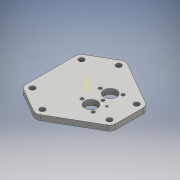
# Autodesk Inventor part: efector
Saved by Autodesk Inventor 2016 SP1 (Build 200210100, 210)
## iProperties
Created: 2016-03-06
Part Number: efector
Material: Generic
Document SubType Name: Modeling
Designer: roduino
Density: 1 g/cm^3
Appearance: Default
Author: roduino
Autodesk Inventor part; units mm, degrees
ref_plane "YZ Plane" through (0, 0, 0) normal (1, 0, 0) x (0, 1, 0)
ref_plane "XZ Plane" through (0, 0, 0) normal (0, 1, 0) x (-1, 0, 0)
ref_plane "XY Plane" through (0, 0, 0) normal (0, 0, 1) x (1, 0, 0)
sketch "Sketch1" plane through (0, 0, 0) normal (0, 0, 1) x (1, 0, 0)
  circle A0 centre (12.9186, 9) radius 6
  circle A1 centre (12.9186, -9) radius 6
  circle A2 centre (-28, 23) radius 2.5
  circle A3 centre (-28, -23) radius 2.5
  arc A4 (-31.4115, -18.0643) -> (-23.8208, -27.3051) centre (-28, -23) ccw
  arc A5 (-23.8208, 27.3051) -> (-31.4115, 18.0643) centre (-28, 23) ccw
  line L0 (-28, 23) -> (-28, -23) construction
  circle A6 centre (0, 0) radius 36.2353 construction
  arc A7 (-11.7365, -34.282) -> (0.0617, -36.2353) centre (-5.9186, -35.7487) ccw
  circle A8 centre (-5.9186, -35.7487) radius 2.5
  arc A9 (31.3499, -18.171) -> (35.5573, -6.9768) centre (33.9186, -12.7487) ccw
  circle A10 centre (33.9186, -12.7487) radius 2.5
  arc A11 (35.5573, 6.9768) -> (31.3499, 18.171) centre (33.9186, 12.7487) ccw
  circle A12 centre (33.9186, 12.7487) radius 2.5
  arc A13 (0.0617, 36.2353) -> (-11.7365, 34.282) centre (-5.9186, 35.7487) ccw
  circle A14 centre (-5.9186, 35.7487) radius 2.5
  line L1 (33.9186, 12.7487) -> (33.9186, -12.7487) construction
  line L2 (-34, 23) -> (-34, -23)
  line L3 (39.9186, 12.7487) -> (39.9186, -12.7487)
  line L4 (-31, 28.1962) -> (-8.9186, 40.9449)
  line L5 (-2.9186, 40.9449) -> (36.9186, 17.9449)
  line L6 (36.9186, -17.9449) -> (-2.9186, -40.9449)
  line L7 (-31, -28.1962) -> (-8.9186, -40.9449)
  dimension "d0" = 12
  dimension "d1" = 12
  dimension "d4" = 5
  dimension "d5" = 5
  dimension "d6" = 46
  dimension "d7" = 23
  dimension "d8" = 28
  dimension "d9" = 28
  dimension "d10" = 12
  dimension "d11" = 12
  dimension "d15" = 360
  dimension "d42" = 25.4974
  dimension "d43" = 27
  dimension "d44" = 27
  dimension "d45" = 9
  dimension "d46" = 9
  constraints: 29 point on circle, 16 end point, 15 centre point, 8 tangent, 7 coincident, 3 parallel, 1 vertical, 37 other
  measures "d0" diameter of A0
  measures "d1" diameter of A1
  measures "d4" diameter of A2
  measures "d5" diameter of A3
  measures "d6" distance of A3.centre A2.centre
  measures "d7" vertical distance of point (0, 0) A3.centre
  measures "d8" horizontal distance of point (0, 0) A2.centre
  measures "d9" horizontal distance of point (0, 0) A3.centre
  measures "d10" diameter of A4
  measures "d11" diameter of A5
  measures "d42" distance of A9.centre A11.centre
  measures "d43" distance from line of L3 A0.centre
  measures "d44" distance from line of L3 A1.centre
  measures "d45" vertical distance of point (0, 0) A0.centre
  measures "d46" vertical distance of point (0, 0) A1.centre
extrude "Extrusion1" add sketch "Sketch1" along normal blind 5
sketch "Sketch2" plane through (0, 0, 5) normal (0, 0, 1) x (1, 0, 0)
  circle A0 centre (12.9186, 9) radius 6 projected
  circle A1 centre (12.9186, -9) radius 6 projected
  circle A2 centre (15, 0) radius 1.5
  circle A3 centre (4, 8.5) radius 1.5
  circle A4 centre (4, -8.5) radius 1.5
  point P0 (0, 0)
  dimension "d19" = 3
  dimension "d20" = 3
  dimension "d21" = 3
  dimension "d22" = 15
  dimension "d25" = 17
  dimension "d26" = 8.5
  dimension "d47" = 4
  dimension "d48" = 4
  constraints: 3 centre point
  measures "d19" diameter of A2
  measures "d20" diameter of A3
  measures "d21" diameter of A4
  measures "d22" distance of point (0, 0) A2.centre
  measures "d25" distance of A4.centre A3.centre
  measures "d26" vertical distance of point (0, 0) A3.centre
  measures "d47" horizontal distance of point (0, 0) A3.centre
  measures "d48" horizontal distance of point (0, 0) A4.centre
extrude "Extrusion2" cut sketch "Sketch2" against normal through all contours A2 | A3 | A4
sketch "Sketch3" plane through (0, 0, 5) normal (0, 0, 1) x (1, 0, 0)
  circle A0 centre (20, 14) radius 1.5
  circle A1 centre (20, -14) radius 1.5
  point P0 (0, 0)
  dimension "d29" = 3
  dimension "d30" = 3
  dimension "d31" = 28
  dimension "d32" = 20
  dimension "d33" = 14
  dimension "d34" = 20
  constraints: 2 centre point
  measures "d29" diameter of A0
  measures "d30" diameter of A1
  measures "d31" distance of A1.centre A0.centre
  measures "d32" horizontal distance of point (0, 0) A1.centre
  measures "d33" vertical distance of point (0, 0) A1.centre
  measures "d34" horizontal distance of point (0, 0) A0.centre
extrude "Extrusion3" cut sketch "Sketch3" against normal through all
sketch "Sketch6" plane through (0, 0, 5) normal (0, 0, 1) x (1, 0, 0)
  arc A0 (22.75, -18) -> (24.75, -16) centre (22.75, -16) ccw projected
  line L0 (22.75, -18) -> (17.25, -18) projected
  arc A1 (15.25, -16) -> (17.25, -18) centre (17.25, -16) ccw projected
  line L1 (15.25, -16) -> (15.25, 16) projected
  arc A2 (17.25, 18) -> (15.25, 16) centre (17.25, 16) ccw projected
  line L2 (17.25, 18) -> (22.75, 18) projected
  arc A3 (24.75, 16) -> (22.75, 18) centre (22.75, 16) ccw projected
  line L3 (24.75, 16) -> (24.75, -16) projected
  circle A4 centre (20, -14) radius 1.5 projected
  circle A5 centre (20, 14) radius 1.5 projected
  circle A6 centre (21.75, -3) radius 1 projected
  point P0 (0, 0)
extrude "Extrusion5" cut sketch "Sketch6" against normal through all contours A6
equation "\"d1\" = d0"
equation "\"d5\" = d4"
equation "\"d7\" = 0.5 * d6"
equation "\"d9\" = d8"
equation "\"d10\" = d11"
equation "\"d46\" = d45"
equation "\"d26\" = 0.5 * d25"
equation "\"d48\" = d47"
equation "\"d33\" = 0.5 * d31"
equation "\"d34\" = d32"
body "Solid1"
